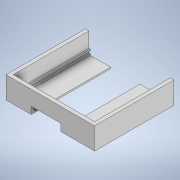
# Autodesk Inventor part: case
Saved by Autodesk Inventor 2022 (Build 260153000, 153)
## iProperties
Created: 2022-04-19
Part Number: case
Material: Generic
Document SubType Name: Modeling
Designer: khonsu
Density: 1 g/cm^3
Appearance: Default
Author: khonsu
Autodesk Inventor part; units mm, degrees
ref_plane "YZ Plane" through (0, 0, 0) normal (1, 0, 0) x (0, 1, 0)
ref_plane "XZ Plane" through (0, 0, 0) normal (0, 1, 0) x (-1, 0, 0)
ref_plane "XY Plane" through (0, 0, 0) normal (0, 0, 1) x (1, 0, 0)
sketch "Sketch1" plane through (0, 0, 0) normal (0, 1, 0) x (-1, 0, 0)
  line L0 (0, 0) -> (56, 0)
  line L1 (56, 0) -> (56, -50)
  line L2 (56, -50) -> (0, -50)
  line L3 (0, -50) -> (0, 0)
  line L4 (56.2, 0) -> (-0.2, 0)
  line L5 (-0.2, 0) -> (-0.2, -50)
  line L6 (-0.2, -50) -> (56.2, -50)
  line L7 (56.2, -50) -> (56.2, 0)
  line L8 (58.7, 2.5) -> (-2.7, 2.5)
  line L9 (-2.7, 2.5) -> (-2.7, -52.5)
  line L10 (-2.7, -52.5) -> (58.7, -52.5)
  line L11 (58.7, -52.5) -> (58.7, 2.5)
  line L12 (56.2, -48.0985) -> (56.2, -52.5)
  line L13 (-0.2, -48.7936) -> (-0.2, -52.5)
  point P0 (-0.2, -50)
  dimension "d0" = 56
  dimension "d1" = 50
  dimension "d2" = 0.2
  dimension "d3" = 0.2
  dimension "d4" = 0
  dimension "d5" = 0
  dimension "d6" = 2.5
  dimension "d7" = 2.5
  dimension "d8" = 2.5
  dimension "d9" = 2.5
  constraints: 28 end point, 6 parallel, 6 point on line, 3 horizontal, 3 perpendicular
  measures "d0" distance of L1.end L2.end
  measures "d1" distance of L0.end L1.end
  measures "d2" distance between parallel lines of L1 L7
  measures "d3" distance between parallel lines of L3 L5
  measures "d4" distance between parallel lines of L0 L4
  measures "d5" distance between parallel lines of L2 L6
  measures "d6" distance between parallel lines of L7 L11
  measures "d7" distance between parallel lines of L0 L8
  measures "d8" distance between parallel lines of L2 L10
  measures "d9" distance between parallel lines of L5 L9
extrude "Extrusion1" add sketch "Sketch1" along normal blind 15.2 contours L4 L5 L13 L10 L9 L8 L11 L12 L7 L0
extrude "Extrusion2" add sketch "Sketch1" along normal blind 1
sketch "Sketch2" plane through (0.2, 15.2, 0) normal (0, 0, -1) x (-1, 0, 0)
  line L0 (0, -14.2) -> (0, 0) projected
  line L1 (0, -13.2) -> (56.4, -13.2)
  line L2 (56.4, -13.2) -> (56.4, -14.2)
  line L3 (56.4, -14.2) -> (0, -14.2)
  line L4 (0, -14.2) -> (0, -13.2)
  line L5 (56.4, -14.2) -> (56.4, 0) projected
  line L6 (0, -14.2) -> (56.4, -14.2) projected
  line L7 (1, -13.2) -> (55.4, -13.2)
  line L8 (55.4, -13.2) -> (55.4, -14.2)
  line L9 (55.4, -14.2) -> (1, -14.2)
  line L10 (1, -14.2) -> (1, -13.2)
  line L11 (0, -10.5) -> (56.4, -10.5)
  line L12 (56.4, -10.5) -> (56.4, -11.5)
  line L13 (56.4, -11.5) -> (0, -11.5)
  line L14 (0, -11.5) -> (0, -10.5)
  line L15 (56.4, -10.5) -> (55.4, -10.5)
  line L16 (55.4, -10.5) -> (55.4, -11.5)
  line L17 (55.4, -11.5) -> (56.4, -11.5)
  line L18 (56.4, -11.5) -> (56.4, -10.5)
  line L19 (0, -10.5) -> (1, -10.5)
  line L20 (1, -10.5) -> (1, -11.5)
  line L21 (1, -11.5) -> (0, -11.5)
  line L22 (0, -11.5) -> (0, -10.5)
  point P0 (0.2, -15.2)
  point P1 (0, -11.5)
  point P2 (1, -14.2)
  dimension "d14" = 0
  dimension "d16" = 1
  dimension "d17" = 1
  dimension "d18" = 1
  dimension "d19" = 0
  dimension "d20" = 0
  dimension "d21" = 1.7
  dimension "d22" = 1
  constraints: 40 end point, 10 parallel, 6 point on line, 5 horizontal, 5 perpendicular
  measures "d14" distance between parallel lines of L5 L2
  measures "d16" distance of L1.end L2.end
  measures "d17" distance between parallel lines of L0 L10
  measures "d18" distance between parallel lines of L5 L8
  measures "d19" distance between parallel lines of L6 L3
  measures "d20" distance between parallel lines of L5 L12
  measures "d21" distance between parallel lines of L7 L13
  measures "d22" distance between parallel lines of L13 L11
extrude "Extrusion3" add sketch "Sketch2" along normal up to surface (52.5 mm away) contours L0 L1 L10 L3 | L0 L11 L20 L13 | L8 L1 L2 L3 | L16 L11 L5 L13
sketch "Sketch3" plane through (2.7, 0, -52.5) normal (0, 0, -1) x (-1, 0, 0)
  line L0 (2.5, 15.2) -> (58.9, 15.2) projected
  line L1 (23.5, 15.2) -> (43.9, 15.2)
  line L2 (43.9, 15.2) -> (43.9, 0)
  line L3 (43.9, 0) -> (23.5, 0)
  line L4 (23.5, 0) -> (23.5, 15.2)
  line L5 (58.9, 4.7) -> (58.9, 15.2) projected
  line L6 (2.5, 4.7) -> (2.5, 15.2) projected
  line L7 (0, 0) -> (61.4, 0) projected
  line L8 (23.5, 0) -> (43.9, 0)
  line L9 (43.9, 0) -> (43.9, 5)
  line L10 (43.9, 5) -> (23.5, 5)
  line L11 (23.5, 5) -> (23.5, 0)
  point P0 (2.7, 0)
  dimension "d25" = 15
  dimension "d26" = 21
  dimension "d27" = 0
  dimension "d30" = 5
  constraints: 16 end point, 4 parallel, 2 horizontal, 2 perpendicular, 2 point on line
  measures "d25" distance between parallel lines of L5 L2
  measures "d26" distance between parallel lines of L6 L4
  measures "d27" distance between parallel lines of L7 L3
  measures "d30" distance of L9.end L8.end
extrude "Extrusion5" cut sketch "Sketch3" against normal blind 75.725 contours L10 L2 L3 L4
equation "\"d23\" = d16"
body "Solid1"
